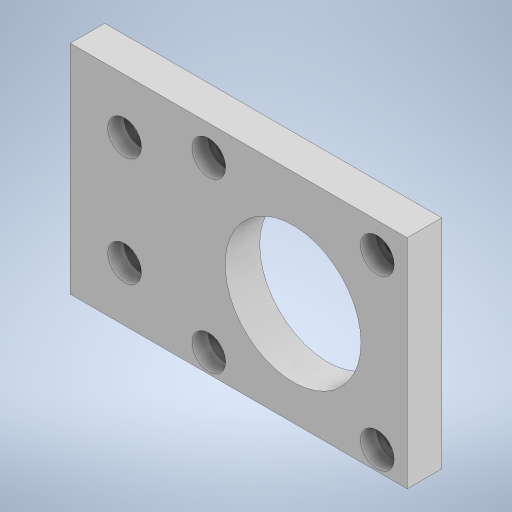
# Autodesk Inventor part: Y Motor Mount
Saved by Autodesk Inventor 2023.1 (Build 271208000, 208)
## iProperties
Created: 2022-11-03
Part Number: Y Motor Mount
Material: Generic
Document SubType Name: Modeling
Designer: nicol
Density: 1 g/cm^3
Appearance: Default
Author: nicol
Autodesk Inventor part; units mm, degrees
ref_plane "YZ Plane" through (0, 0, 0) normal (1, 0, 0) x (0, 1, 0)
ref_plane "XZ Plane" through (0, 0, 0) normal (0, 1, 0) x (-1, 0, 0)
ref_plane "XY Plane" through (0, 0, 0) normal (0, 0, 1) x (1, 0, 0)
sketch "Sketch1" plane through (0, 0, 0) normal (0, 0, 1) x (1, 0, 0)
  line L0 (0, 0) -> (62, 0)
  line L1 (62, 0) -> (62, 40)
  line L2 (62, 40) -> (0, 40)
  line L3 (0, 40) -> (0, 0)
  line L4 (20, 40) -> (62, 40) construction
  line L5 (62, 40) -> (62, -2) construction
  line L6 (62, -2) -> (20, -2) construction
  line L7 (20, -2) -> (20, 40) construction
  line L8 (25.5, 34.5) -> (56.5, 34.5) construction
  line L9 (56.5, 34.5) -> (56.5, 3.5) construction
  line L10 (56.5, 3.5) -> (25.5, 3.5) construction
  line L11 (25.5, 3.5) -> (25.5, 34.5) construction
  point P0 (25.5, 19)
  point P1 (20, 19)
  point P2 (41, 34.5)
  point P3 (41, 40)
  point P4 (41, 19)
  point P5 (10, 30)
  point P6 (10, 10)
  dimension "d0" = 40
  dimension "d1" = 62
  dimension "d2" = 42
  dimension "d3" = 42
  dimension "d4" = 31
  dimension "d5" = 31
  dimension "d22" = 10
  dimension "d23" = 10
  dimension "d24" = 10
  constraints: 24 end point, 6 parallel, 4 coincident, 4 midpoint, 3 horizontal, 3 perpendicular, 3 vertical alignment, 2 horizontal alignment
  measures "d0" distance of L2.end L0.start
  measures "d1" distance of L1.end L2.end
  measures "d2" distance of L5.end L6.end
  measures "d3" distance of L1.end L5.end
  measures "d4" distance of L9.end L10.end
  measures "d5" distance of L8.end L9.end
  measures "d22" distance from line of L0 point (10, 10)
  measures "d23" distance from line of L2 point (10, 30)
  measures "d24" distance from line of L3 point (10, 10)
extrude "Extrusion1" add sketch "Sketch1" against normal blind 6.35
hole "Hole1" at (25.5, 34.5, 0) at (56.5, 34.5, 0) at (56.5, 3.5, 0) at (25.5, 3.5, 0) at (10, 30, 0) at (10, 10, 0) direction (0, 0, -1) diameter 3.2 end through all counterbore diameter 6.2 counterbore depth 3
hole "Hole2" at (41, 19, 0) direction (0, 0, -1) diameter 25 end through all
body "Solid1"
